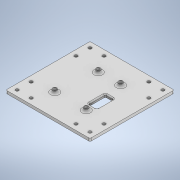
# Autodesk Inventor part: agv_nano_base
Saved by Autodesk Inventor 2021.2 (Build 252289000, 289)
## iProperties
Created: 2021-04-20
Part Number: agv_nano_base
Material: Generic
Document SubType Name: Modeling
Designer: jesse
Density: 1 g/cm^3
Appearance: Default
Author: jesse
Autodesk Inventor part; units mm, degrees
ref_plane "YZ Plane" through (0, 0, 0) normal (1, 0, 0) x (0, 1, 0)
ref_plane "XZ Plane" through (0, 0, 0) normal (0, 1, 0) x (-1, 0, 0)
ref_plane "XY Plane" through (0, 0, 0) normal (0, 0, 1) x (1, 0, 0)
sketch "Sketch2" plane through (0, 0, 0) normal (0, 1, 0) x (-1, 0, 0)
  line L0 (67.9954, 72.8645) -> (-82.0046, 72.8645)
  line L1 (-82.0046, 72.8645) -> (-82.0046, -77.1355)
  line L2 (-82.0046, -77.1355) -> (67.9954, -77.1355)
  line L3 (67.9954, -77.1355) -> (67.9954, 72.8645)
  circle A0 centre (57.9954, 62.8645) radius 2.75
  circle A1 centre (32.9954, 62.8645) radius 2.75
  circle A2 centre (57.9954, 37.8645) radius 2.75
  line L4 (67.9954, -2.1355) -> (-82.0046, -2.1355)
  line L5 (-7.0046, 72.8645) -> (-7.0046, -77.1355)
  circle A3 centre (57.9954, -67.1355) radius 2.75
  circle A4 centre (32.9954, -67.1355) radius 2.75
  circle A5 centre (57.9954, -42.1355) radius 2.75
  circle A6 centre (-72.0046, 62.8645) radius 2.75
  circle A7 centre (-47.0046, 62.8645) radius 2.75
  circle A8 centre (-72.0046, 37.8645) radius 2.75
  circle A9 centre (-72.0046, -67.1355) radius 2.75
  circle A10 centre (-72.0046, -42.1355) radius 2.75
  circle A11 centre (-47.0046, -67.1355) radius 2.75
  point P0 (0, 0)
  dimension "d0" = 150
  dimension "d1" = 150
  dimension "d2" = 10
  dimension "d3" = 10
  dimension "d4" = 25
  dimension "d5" = 25
  dimension "d6" = 10
  dimension "d7" = 10
  dimension "d42" = 5.5
  dimension "d43" = 5.5
  dimension "d44" = 5.5
  constraints: 12 centre point, 12 end point, 9 symmetric about line, 4 midpoint, 2 parallel, 1 horizontal, 1 perpendicular, 9 other
  measures "d0" distance of L2.end L0.start
  measures "d1" distance of L1.end L2.end
  measures "d2" distance from line of L3 A0.centre
  measures "d3" distance from line of A0.centre L0
  measures "d4" distance of A2.centre A0.centre
  measures "d5" distance of A0.centre A1.centre
  measures "d6" distance from line of L0 A1.centre
  measures "d7" distance from line of L3 A2.centre
  measures "d42" diameter of A11
  measures "d43" diameter of A9
  measures "d44" diameter of A10
extrude "Extrusion1" add sketch "Sketch2" along normal blind 5
sketch "Sketch4" plane through (0, 5, 0) normal (0, 1, 0) x (1, 0, 0)
  line L0 (-12.9954, 36.8855) -> (27.0046, 36.8855)
  line L1 (27.0046, 36.8855) -> (35.0046, -32.6145)
  line L2 (35.0046, -32.6145) -> (-20.9954, -32.6145)
  line L3 (-20.9954, -32.6145) -> (-12.9954, 36.8855)
  line L4 (7.0046, 36.8855) -> (7.0046, -32.6145)
  line L5 (82.0046, -72.8645) -> (82.0046, 77.1355) projected
  line L6 (-16.9954, 2.1355) -> (31.0046, 2.1355)
  line L7 (82.0046, 77.1355) -> (-67.9954, 77.1355) projected
  circle A0 centre (-12.9954, 36.8855) radius 2.7
  circle A1 centre (27.0046, 36.8855) radius 2.7
  circle A2 centre (35.0046, -32.6145) radius 2.7
  circle A3 centre (-20.9954, -32.6145) radius 2.7
  circle A4 centre (-12.9954, 36.8855) radius 3.7
  circle A5 centre (27.0046, 36.8855) radius 3.7
  circle A6 centre (35.0046, -32.6145) radius 3.7
  circle A7 centre (-20.9954, -32.6145) radius 3.7
  point P0 (0, 0)
  dimension "d17" = 40
  dimension "d18" = 56
  dimension "d19" = 75
  dimension "d20" = 75
  dimension "d21" = 5.4
  dimension "d22" = 5.4
  dimension "d23" = 5.4
  dimension "d24" = 5.4
  dimension "d25" = 1
  dimension "d26" = 1
  dimension "d27" = 1
  dimension "d28" = 1
  dimension "d45" = 69.5
  constraints: 12 end point, 8 centre point, 8 coincident, 4 midpoint, 1 horizontal, 1 parallel, 1 perpendicular
  measures "d17" distance of L0.start L0.end
  measures "d18" distance of L1.end L2.end
  measures "d19" distance between parallel lines of L5 L4
  measures "d20" distance between parallel lines of L7 L6
  measures "d21" diameter of A0
  measures "d22" diameter of A1
  measures "d23" diameter of A2
  measures "d24" diameter of A3
  measures "d25" radial gap between concentric circles of A4 A0
  measures "d26" radial gap between concentric circles of A5 A1
  measures "d27" radial gap between concentric circles of A6 A2
  measures "d28" radial gap between concentric circles of A7 A3
  measures "d45" distance of L4.start L4.end
extrude "Extrusion3" add sketch "Sketch4" along normal blind 5 contours A0 L3 A4 L0 | L0 A4 L3 A0 | A5 L1 A1 L0 | L0 A1 L1 A5 | A7 L2 A3 L3 | L3 A3 L2 A7 | A6 L1 A2 L2 | L2 A2 L1 A6
sketch "Sketch5" plane through (-20.9954, 5, 32.6145) normal (0, 1, 0) x (1, 0, 0)
  circle A0 centre (0, 0) radius 2.7 projected
  circle A1 centre (0, 0) radius 2.7
  circle A2 centre (48, 69.5) radius 2.7 projected
  circle A3 centre (48, 69.5) radius 2.7
  circle A4 centre (56, 0) radius 2.7 projected
  circle A5 centre (56, 0) radius 2.7
  circle A6 centre (8, 69.5) radius 3.7 projected
  circle A7 centre (8, 69.5) radius 2.7
  point P0 (20.9954, 32.6145)
  constraints: 4 centre point, 4 coincident
extrude "Extrusion4" cut sketch "Sketch5" against normal through all contours A0 | A2 | A4 | A7
fillet "Fillet1" radius 4 4 edges at (-24.6954, 5, 32.6145) (31.3046, 5, 32.6145) (23.3046, 5, -36.8855) (-16.6954, 5, -36.8855)
sketch "Sketch6" plane through (0, 5, 0) normal (0, 1, 0) x (1, 0, 0)
  line L0 (26.5046, 9.8855) -> (41.5046, 9.8855)
  line L1 (41.5046, 9.8855) -> (41.5046, -20.1145)
  line L2 (41.5046, -20.1145) -> (26.5046, -20.1145)
  line L3 (26.5046, -20.1145) -> (26.5046, 9.8855)
  line L4 (26.5046, -5.1145) -> (41.5046, -5.1145)
  line L5 (34.0046, 9.8855) -> (34.0046, -20.1145)
  circle A0 centre (35.0046, -32.6145) radius 2.7 projected
  point P0 (0, 0)
  dimension "d34" = 15
  dimension "d35" = 30
  dimension "d36" = 27.5
  dimension "d37" = 1
  constraints: 12 end point, 4 midpoint, 2 parallel, 1 horizontal, 1 perpendicular
  measures "d34" distance of L0.start L0.end
  measures "d35" distance of L0.end L1.end
  measures "d36" distance from line of A0.centre L4
  measures "d37" distance from line of A0.centre L5
extrude "Extrusion5" cut sketch "Sketch6" against normal through all contours L0 L5 L4 L3 | L0 L1 L4 L5 | L4 L5 L2 L3 | L4 L1 L2 L5
fillet "Fillet3" radius 2.5 4 edges at (-67.9954, 2.5, 72.8645) (82.0046, 2.5, 72.8645) (82.0046, 2.5, -77.1355) (-67.9954, 2.5, -77.1355)
fillet "Fillet4" radius 2 8 edges at (41.5046, 2.5, -9.8855) (41.5046, 5, 5.1145) (34.0046, 5, -9.8855) (26.5046, 2.5, -9.8855) (26.5046, 5, 5.1145) (34.0046, 5, 20.1145) (26.5046, 2.5, 20.1145) (41.5046, 2.5, 20.1145)
equation "\"d1\" = d0"
equation "\"d6\" = d3"
equation "\"d7\" = d2"
equation "\"d22\" = d21"
equation "\"d23\" = d21"
equation "\"d24\" = d21"
equation "\"d26\" = d25"
equation "\"d27\" = d25"
equation "\"d28\" = d25"
body "Solid1"
